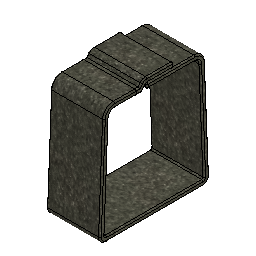
BatteryStrap v2 (Autodesk Fusion 360 design; units mm, degrees)
Autodesk Fusion 360 part; units mm, degrees
sketch "Sketch9" plane through (0, 0, 0) normal (0, 0, 1) x (1, 0, 0)
  line L0 (-37.5, 17) -> (37.5, 17) construction
  line L1 (37.5, 17) -> (37.5, -17) construction
  line L2 (37.5, -17) -> (-37.5, -17) construction
  line L3 (-37.5, -17) -> (-37.5, 17) construction
  line L4 (-37.5, 0) -> (37.5, 0) construction
  line L5 (-12.5, 21) -> (7.5, 21) construction
  line L6 (7.5, 18) -> (-12.5, 18) construction
  arc A0 (-12.5, 21) -> (-12.5, 18) centre (-12.5, 19.5) ccw construction
  arc A1 (7.5, 18) -> (7.5, 21) centre (7.5, 19.5) ccw construction
  arc A2 (-12.5, -18) -> (-12.5, -21) centre (-12.5, -19.5) ccw construction
  line L7 (7.5, -18) -> (-12.5, -18) construction
  line L8 (-12.5, -21) -> (7.5, -21) construction
  arc A3 (7.5, -21) -> (7.5, -18) centre (7.5, -19.5) ccw construction
  point P0 (-37.5, 0)
  point P1 (37.5, 0)
  dimension "d147" = 75
  dimension "d148" = 34
  dimension "d151" = 3
  dimension "d152" = 20
  dimension "d153" = 1
  dimension "d154" = 30
  dimension "d155" = 1.5
  constraint horizontal L0
  constraint vertical L1
  constraint horizontal L2
  constraint vertical L3
  constraint midpoint L3 P0
  constraint midpoint L1 P1
  constraint coincident P0 L4.start
  constraint coincident P1 L4.end
  constraint midpoint L4 origin
  constraint parallel L0 L5
  constraint parallel L5 L6
  constraint tangent L5 A0
  constraint tangent L6 A1
  constraint tangent L5 A1
  constraint symmetric L4 L5.start A2.end
  constraint symmetric L4 L5.end L8.end
  constraint symmetric L4 L6.start L7.start
  constraint symmetric L4 L6.end A2.start
  constraint symmetric L4 A0 A2
  constraint symmetric L4 A1 A3
  measures "d147" distance of L0.start L0.end
  measures "d148" distance of L0.start L2.end
  measures "d151" distance of L5 L6
  measures "d152" distance of L5.start L5.end
  measures "d153" distance of L0 L6
  measures "d154" distance of L1 L5.end
  measures "d155" radius of A0
ref_plane "WorkPlane7" through (0, 0, -4.3) normal (0, 0, 1) x (1, 0, 0)
sketch "Sketch10" plane through (0, 0, -4.3) normal (0, 0, 1) x (1, 0, 0)
  line L0 (7.5, 18) -> (-12.5, 18)
  arc A0 (-12.5, 21) -> (-12.5, 18) centre (-12.5, 19.5) ccw
  line L1 (-12.5, 21) -> (7.5, 21)
  arc A1 (7.5, 18) -> (7.5, 21) centre (7.5, 19.5) ccw
  line L2 (-12.5, 20.5) -> (7.5, 20.5)
  line L3 (7.5, 20.5) -> (7.5, 18.5)
  line L4 (7.5, 18.5) -> (-12.5, 18.5)
  line L5 (-12.5, 18.5) -> (-12.5, 20.5)
  point P0 (7.5, 19.5)
  dimension "d157" = 2
  dimension "d158" = 0.5
  dimension "d159" = 20
  constraint horizontal L2
  constraint vertical L3
  constraint horizontal L4
  constraint vertical L5
  constraint coincident L3 P0
  measures "d157" distance of L2.start L4.end
  measures "d158" distance of L0 L4
  measures "d159" distance of L2.start L2.end
ref_plane "WorkPlane8" through (7.5, 0, 0) normal (1, 0, 0) x (0, 1, 0)
sketch "Sketch11" plane through (7.5, 0, 0) normal (1, 0, 0) x (0, 1, 0)
  line L0 (-18, 0) -> (-21, 0)
  line L1 (21, -4.3) -> (18, -4.3)
  line L2 (-15, 0) -> (15, 0) construction
  line L3 (17, 2) -> (17, 33) construction
  line L4 (15, 35) -> (-15, 35) construction
  line L5 (-17, 33) -> (-17, 2) construction
  line L6 (-15, 33) -> (15, 33) construction
  line L7 (15, 33) -> (15, 2) construction
  line L8 (15, 2) -> (-15, 2) construction
  line L9 (-15, 2) -> (-15, 33) construction
  line L10 (17, 0) -> (-17, 0) construction
  circle A0 centre (15, 2) radius 2 construction
  circle A1 centre (-15, 2) radius 2 construction
  line L11 (18, 0) -> (21, 0) construction
  line L12 (21, 0) -> (21, -4.8) construction
  line L13 (21, -4.8) -> (18, -4.8) construction
  line L14 (18, -4.8) -> (18, 0) construction
  line L15 (-18, -4.8) -> (-21, -4.8) construction
  line L16 (-21, -4.8) -> (-21, 0) construction
  line L17 (-21, 0) -> (-18, 0) construction
  line L18 (-18, 0) -> (-18, -4.8) construction
  arc A2 (18, -4.8) -> (18.4996, -4.2799) centre (18, -4.3) ccw
  line L19 (20.5, -4.3) -> (18.5, -4.3)
  arc A3 (-18.4996, -4.2799) -> (-18, -4.8) centre (-18, -4.3) ccw
  line L20 (-18, -4.3) -> (-18.5, -4.3) construction
  line L21 (-18, -4.3) -> (-18, -4.8) construction
  line L22 (-18, -4.8) -> (18, -4.8)
  line L23 (18.4996, -4.2799) -> (16.9984, 33.0803)
  line L24 (-18.4996, -4.2799) -> (-16.9984, 33.0803)
  line L25 (-15, 35) -> (-7, 35)
  line L26 (15, 35) -> (-3, 35)
  arc A4 (-16.9984, 33.0803) -> (-15, 35) centre (-15, 33) ccw construction
  arc A5 (-15, 35) -> (-16.9984, 33.0803) centre (-15, 33) ccw
  arc A6 (15, 35) -> (16.9984, 33.0803) centre (15, 33) ccw construction
  arc A7 (16.9984, 33.0803) -> (15, 35) centre (15, 33) ccw
  point P0 (19.5, 0)
  point P1 (-19.5, 0)
  point P2 (-18, -4.3)
  dimension "d165" = 2
  dimension "d166" = 2
  dimension "d167" = 2
  dimension "d168" = 2
  dimension "d169" = 34
  dimension "d170" = 35
  dimension "d171" = 3
  dimension "d172" = 4.8
  dimension "d173" = 3
  dimension "d174" = 4.8
  dimension "d175" = 0.5
  dimension "d176" = 90
  dimension "d177" = 8
  dimension "d178" = 18
  constraint horizontal L2
  constraint vertical L3
  constraint horizontal L4
  constraint vertical L5
  constraint horizontal L6
  constraint vertical L7
  constraint horizontal L8
  constraint vertical L9
  constraint coincident L6.start L9.end
  constraint tangent L4 A4
  constraint coincident L6.end L7.start
  constraint tangent L4 A6
  constraint coincident L7.end L8.start
  constraint tangent L3 A0
  constraint coincident L8.end L9.start
  constraint tangent L5 A1
  constraint coincident L5.start A4
  constraint coincident L3.end A6
  constraint coincident A0 L3.start
  constraint coincident A0 L2.end
  constraint coincident A1 L2.start
  constraint coincident A1 L5.end
  constraint midpoint L2 origin
  constraint horizontal L11
  constraint vertical L12
  constraint horizontal L13
  constraint vertical L14
  constraint coincident L1.end L14
  constraint coincident L11 P0
  constraint horizontal L15
  constraint vertical L16
  constraint horizontal L17
  constraint vertical L18
  constraint coincident L17 P1
  constraint coincident L0.start L17.end
  constraint coincident L18 P2
  constraint coincident L1.end A2.centre
  constraint coincident P2 A3.centre
  constraint tangent L23 A6
  constraint tangent A2 L23
  constraint tangent L24 A4
  constraint tangent A3 L24
  constraint coincident L20.end A3
  constraint parallel L4 L25
  constraint tangent L26 A6
  constraint concentric A4 A5
  constraint concentric A6 A7
  measures "d165" distance of L4 L6
  measures "d166" distance of L5 L9
  measures "d167" distance of L3 L7
  measures "d168" distance of L8 L10
  measures "d169" distance of L3 L5
  measures "d170" distance of L4 L10
  measures "d171" distance of L11.start L11.end
  measures "d172" distance of L11.start L13.end
  measures "d173" distance of L15.start L15.end
  measures "d174" distance of L15.start L0.start
  measures "d175" distance of L15 P2
  measures "d176" angle of L20 L21
  measures "d177" distance of L4.end L25.end
  measures "d178" distance of L4.start L26.end
sketch "Sketch12" plane through (7.5, 0, 0) normal (1, 0, 0) x (0, 1, 0)
  line L0 (-3, 35) -> (-3, 37) construction
  line L1 (-3, 37) -> (7, 37)
  line L2 (-7, 35) -> (-5, 35)
  line L3 (-5, 35) -> (-5, 35.5) construction
  line L4 (-3.4, 36.8) -> (-4.6, 35.2)
  arc A0 (-5, 35) -> (-4.6, 35.2) centre (-5, 35.5) ccw
  arc A1 (-4.6, 35.2) -> (-5, 35) centre (-5, 35.5) ccw construction
  arc A2 (-3.4, 36.8) -> (-3, 37) centre (-3, 36.5) ccw construction
  arc A3 (-3, 37) -> (-3.4, 36.8) centre (-3, 36.5) ccw
  point P0 (-3, 35)
  point P1 (-3, 36.5)
  point P2 (-7, 35)
  dimension "d181" = 2
  dimension "d182" = 10
  dimension "d183" = 0.5
  dimension "d184" = 2
  dimension "d185" = 0.5
  constraint coincident P0 L0.start
  constraint vertical L0
  constraint perpendicular L0 L1
  constraint coincident L0 P1
  constraint coincident P1 A2.centre
  constraint coincident P2 L2.start
  constraint horizontal L2
  constraint perpendicular L2 L3
  constraint coincident L3.end A0.centre
  constraint tangent L4 A0
  constraint tangent L4 A2
  constraint concentric A0 A1
  constraint concentric A2 A3
  measures "d181" distance of P0 L0.end
  measures "d182" distance of L0.end L1.end
  measures "d183" distance of L1 P1
  measures "d184" distance of P2 L2.end
  measures "d185" distance of L2.end L3.end
ref_plane "WorkPlane9" through (0, 7, 0) normal (0, 1, 0) x (0, 0, 1)
sketch "Sketch13" plane through (0, 7, 0) normal (0, 1, 0) x (1, 0, 0)
  line L0 (-12.5, -39) -> (7.5, -39)
  line L1 (7.5, -39) -> (7.5, -37)
  line L2 (7.5, -37) -> (-12.5, -37)
  line L3 (-12.5, -37) -> (-12.5, -39)
  point P0 (7.5, -37)
  dimension "d187" = 20
  dimension "d188" = 2
  constraint horizontal L0
  constraint vertical L1
  constraint horizontal L2
  constraint vertical L3
  constraint coincident P0 L1.end
  measures "d187" distance of L0.start L0.end
  measures "d188" distance of L0.start L2.end
sweep "Sweep6" add profiles "Sketch10" path "Sketch11" along L25 A5 L24 A3 L22 A2 L23 A7 L26 section 1 contours L2 L3 L4 L5 makes body 1
sweep "Sweep7" add profiles "Sketch13" path "Sketch12" along L2 A0 L4 A3 L1 section 1 separate body makes body 2
fillet "Fillet8" radius 0.5 62 edges at (7.5, 6, 37) (7.5, 17.7711, 35.8846) (7.5, 19.7474, 14.4805) (7.5, 19.8029, -6.0319) (7.5, 0, -6.8) (7.5, -19.8029, -6.0319) (7.5, -19.7474, 14.4805) (7.5, -17.7711, 35.8846) (7.5, -11, 37) (7.5, 6, 35) (7.5, 16.3855, 34.4423) (7.5, 17.749, 14.4002) (7.5, 18.3606, -4.6464) (7.5, 0, -4.8) (7.5, -18.3606, -4.6464) (7.5, -17.749, 14.4002) (7.5, -16.3855, 34.4423) (7.5, -11, 35) (-12.5, 6, 37) (-12.5, 17.7711, 35.8846) (-12.5, 19.7474, 14.4805) (-12.5, 19.8029, -6.0319) (-12.5, 0, -6.8) (-12.5, -19.8029, -6.0319) (-12.5, -19.7474, 14.4805) (-12.5, -17.7711, 35.8846) (-12.5, -11, 37) (-12.5, 6, 35) (-12.5, 16.3855, 34.4423) (-12.5, 17.749, 14.4002) (-12.5, 18.3606, -4.6464) (-12.5, 0, -4.8) (-12.5, -18.3606, -4.6464) (-12.5, -17.749, 14.4002) (-12.5, -16.3855, 34.4423) (-12.5, -11, 35) (-2.5, -3, 35) (7.5, -3, 36) (-2.5, -3, 37) (-12.5, -3, 36) (-12.5, 2, 39) (-12.5, -4.118, 38.7361) (-12.5, -5.375, 37.5) (7.5, 2, 39) (7.5, -4.118, 38.7361) (7.5, -5.375, 37.5) (-2.5, 7, 39) (-2.5, 7, 37) (7.5, 7, 38) (-12.5, 7, 38) (-12.5, -6.375, 37) (7.5, -6.375, 37) (7.5, 2, 37) (7.5, -3.2236, 36.9472) (7.5, -4, 36) (7.5, -4.7764, 35.0528) (7.5, -6, 35) (-12.5, 2, 37) (-12.5, -3.2236, 36.9472) (-12.5, -4, 36) (-12.5, -4.7764, 35.0528) (-12.5, -6, 35) on bodies 1 2
